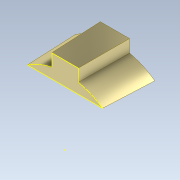
# Autodesk Inventor part: Capstonradialdisc_Aufmass
Saved by Autodesk Inventor 2022 (Build 260153000, 153)
## iProperties
Created: 2022-03-11
Part Number: Capstonradialdisc_Aufmass
Material: Generisch
Document SubType Name: Modeling
Designer: 123St
Density: 1 g/cm^3
Appearance: Gold - Metall
Author: 123St
Autodesk Inventor part; units mm, degrees
ref_plane "YZ Plane" through (0, 0, 0) normal (1, 0, 0) x (0, 1, 0)
ref_plane "XZ Plane" through (0, 0, 0) normal (0, 1, 0) x (-1, 0, 0)
ref_plane "XY Plane" through (0, 0, 0) normal (0, 0, 1) x (1, 0, 0)
sketch "Skizze1" plane through (0, 0, 0) normal (0, 0, 1) x (1, 0, 0)
  line L0 (-4, 23.3) -> (4, 23.3)
  line L1 (4, 23.3) -> (4, 20)
  line L2 (-4, 20) -> (-4, 23.3)
  line L3 (-4, 23.3) -> (4, 20) construction
  line L4 (4, 23.3) -> (-4, 20) construction
  line L5 (0, 152) -> (0, -72) projected
  line L6 (4, 20) -> (4, 19.5959)
  line L7 (-4, 20) -> (-4, 19.5959)
  arc A0 (-4, 19.5959) -> (4, 19.5959) centre (0, 0) ccw
  line L8 (-168, 0) -> (168, 0) projected
  line L9 (-35, 0) -> (-105, 0) construction
  line L10 (-35, -3) -> (-105, -3)
  line L11 (-105, 3) -> (-35, 3)
  arc A1 (-35, -3) -> (-35, 3) centre (-35, 0) ccw
  arc A2 (-105, 3) -> (-105, -3) centre (-105, 0) ccw
  arc A3 (-38.9589, -9.0666) -> (38.9589, -9.0666) centre (0, 0) ccw
  line L12 (-38.9589, -9.0666) -> (-119.657, -9.0666)
  line L13 (38.9589, -9.0666) -> (119.657, -9.0666)
  arc A4 (119.657, -9.0666) -> (-119.657, -9.0666) centre (0, 0) ccw
  arc A5 (-33.4838, 10.6223) -> (-31.1877, 16.1656) centre (-32.3358, 13.3939) ccw
  line L14 (-95.8593, 42.9534) -> (-31.1877, 16.1656)
  line L15 (-32.3358, 13.3939) -> (-97.0074, 40.1818) construction
  arc A6 (-95.8593, 42.9534) -> (-98.1554, 37.4101) centre (-97.0074, 40.1818) ccw
  line L16 (-33.4838, 10.6223) -> (-98.1554, 37.4101)
  arc A7 (-26.8701, 22.6274) -> (-22.6274, 26.8701) centre (-24.7487, 24.7487) ccw
  line L17 (-72.1249, 76.3675) -> (-22.6274, 26.8701)
  line L18 (-24.7487, 24.7487) -> (-74.2462, 74.2462) construction
  arc A8 (-72.1249, 76.3675) -> (-76.3675, 72.1249) centre (-74.2462, 74.2462) ccw
  line L19 (-26.8701, 22.6274) -> (-76.3675, 72.1249)
  arc A9 (-16.1656, 31.1877) -> (-10.6223, 33.4838) centre (-13.3939, 32.3358) ccw
  line L20 (-37.4101, 98.1554) -> (-10.6223, 33.4838)
  line L21 (-13.3939, 32.3358) -> (-40.1818, 97.0074) construction
  arc A10 (-37.4101, 98.1554) -> (-42.9534, 95.8593) centre (-40.1818, 97.0074) ccw
  line L22 (-16.1656, 31.1877) -> (-42.9534, 95.8593)
  arc A11 (-3, 35) -> (3, 35) centre (0, 35) ccw
  line L23 (3, 105) -> (3, 35)
  line L24 (0, 35) -> (0, 105) construction
  arc A12 (3, 105) -> (-3, 105) centre (0, 105) ccw
  line L25 (-3, 35) -> (-3, 105)
  arc A13 (10.6223, 33.4838) -> (16.1656, 31.1877) centre (13.3939, 32.3358) ccw
  line L26 (42.9534, 95.8593) -> (16.1656, 31.1877)
  line L27 (13.3939, 32.3358) -> (40.1818, 97.0074) construction
  arc A14 (42.9534, 95.8593) -> (37.4101, 98.1554) centre (40.1818, 97.0074) ccw
  line L28 (10.6223, 33.4838) -> (37.4101, 98.1554)
  arc A15 (22.6274, 26.8701) -> (26.8701, 22.6274) centre (24.7487, 24.7487) ccw
  line L29 (76.3675, 72.1249) -> (26.8701, 22.6274)
  line L30 (24.7487, 24.7487) -> (74.2462, 74.2462) construction
  arc A16 (76.3675, 72.1249) -> (72.1249, 76.3675) centre (74.2462, 74.2462) ccw
  line L31 (22.6274, 26.8701) -> (72.1249, 76.3675)
  arc A17 (31.1877, 16.1656) -> (33.4838, 10.6223) centre (32.3358, 13.3939) ccw
  line L32 (98.1554, 37.4101) -> (33.4838, 10.6223)
  line L33 (32.3358, 13.3939) -> (97.0074, 40.1818) construction
  arc A18 (98.1554, 37.4101) -> (95.8593, 42.9534) centre (97.0074, 40.1818) ccw
  line L34 (31.1877, 16.1656) -> (95.8593, 42.9534)
  arc A19 (35, 3) -> (35, -3) centre (35, 0) ccw
  line L35 (105, -3) -> (35, -3)
  line L36 (35, 0) -> (105, 0) construction
  arc A20 (105, -3) -> (105, 3) centre (105, 0) ccw
  line L37 (35, 3) -> (105, 3)
  line L38 (-55.3007, 11) -> (-101.4947, 30.1342)
  line L39 (-101.4947, 30.1342) -> (-105.3007, 11)
  line L40 (-105.3007, 11) -> (-55.3007, 11)
  line L41 (-82.1538, 66.7832) -> (-93.0127, 50.5755)
  line L42 (-46.8426, 31.3838) -> (-82.1538, 66.7832)
  line L43 (-93.0127, 50.5755) -> (-46.8426, 31.3838)
  line L44 (-50.2273, 93.2012) -> (-66.4754, 82.403)
  line L45 (-31.2084, 46.9597) -> (-50.2273, 93.2012)
  line L46 (-66.4754, 82.403) -> (-31.2084, 46.9597)
  line L47 (-10.6061, 105.3411) -> (-29.7544, 101.6067)
  line L48 (-10.7931, 55.3415) -> (-10.6061, 105.3411)
  line L49 (-29.7544, 101.6067) -> (-10.7931, 55.3415)
  line L50 (30.6399, 101.3432) -> (11.525, 105.2446)
  line L51 (11.2756, 55.2452) -> (30.6399, 101.3432)
  line L52 (11.525, 105.2446) -> (11.2756, 55.2452)
  line L53 (67.192, 81.8198) -> (51.0387, 92.7593)
  line L54 (31.617, 46.6855) -> (67.192, 81.8198)
  line L55 (51.0387, 92.7593) -> (31.617, 46.6855)
  line L56 (93.4505, 49.7619) -> (82.7335, 66.0637)
  line L57 (47.1147, 30.9738) -> (93.4505, 49.7619)
  line L58 (82.7335, 66.0637) -> (47.1147, 30.9738)
  line L59 (105.3927, 10.0807) -> (101.7538, 29.2473)
  line L60 (55.3946, 10.517) -> (105.3927, 10.0807)
  line L61 (101.7538, 29.2473) -> (55.3946, 10.517)
  point P0 (0, 21.65)
  point P1 (-70, 0)
  point P2 (-64.6716, 26.7878)
  point P3 (-49.4975, 49.4975)
  point P4 (-26.7878, 64.6716)
  point P5 (0, 70)
  point P6 (26.7878, 64.6716)
  point P7 (49.4975, 49.4975)
  point P8 (64.6716, 26.7878)
  point P9 (70, 0)
  dimension "d2" = 8
  dimension "d3" = 0
  dimension "d4" = 3.3
  dimension "d7" = 70
  dimension "d8" = 3
  dimension "d9" = 70
  dimension "d12" = 180
  dimension "d18" = 120
  dimension "d19" = 40
  dimension "d21" = 8
  dimension "d22" = 8
  dimension "d23" = 50
  dimension "d24" = 50
  dimension "d27" = 158
  constraints: 138 end point, 42 point on circle, 21 centre point, 5 parallel, 4 coincident, 4 point on line, 4 tangent, 3 midpoint, 2 horizontal, 1 perpendicular, 1 vertical, 147 other
  measures "d2" distance of L0.start L0.end
  measures "d3" distance from line of L5 point (0, 21.65)
  measures "d4" distance of L0.end L1.end
  measures "d7" distance of L11.start L11.end
  measures "d8" radius of A1
  measures "d9" distance of point (0, 0) point (-70, 0)
  measures "d18" radius of A4
  measures "d19" radius of A3
  measures "d21" distance between parallel lines of L11 L40
  measures "d22" distance between parallel lines of L16 L38
  measures "d23" distance of L39.end L38.start
  measures "d24" distance of L38.start L38.end
extrude "Extrusion1" add sketch "Skizze1" along normal blind 15 contours L2 L7 A0 L8 A1 L11 A2 A4 L5 A12 L25 A11 L0 | L5 A11 L23 A12 A4 L8 A20 L37 A19 A0 L6 L1 L0 | A0 L8 A19 L35 A20 A4 L13 A3 L5 | L5 A3 L12 A4 L8 A2 L10 A1 A0
fillet "Rundung1" radius 15 2 edges at (-38.9589, -9.0666, 7.5) (38.9589, -9.0666, 7.5)
fillet "Rundung2" radius 5 2 edges at (119.657, -9.0666, 7.5) (-119.657, -9.0666, 7.5)
sketch "Skizze2" plane through (49.455, -9.0666, 0) normal (0, -1, 0) x (1, 0, 0)
  circle A0 centre (62.4699, 2.5) radius 1
  line L0 (0, 0) -> (65.4731, 0) projected
  circle A1 centre (-161.38, 12.5) radius 1
  line L1 (-164.3831, 15) -> (-98.91, 15) projected
  line L2 (-169.38, 15) -> (-169.38, 0) projected
  line L3 (70.4699, 0) -> (70.4699, 15) projected
  point P0 (-49.455, 0)
  dimension "d29" = 2.5
  dimension "d30" = 2
  dimension "d31" = 2.5
  dimension "d32" = 2
  dimension "d33" = 8
  dimension "d34" = 8
  constraints: 2 centre point
  measures "d29" distance from line of L0 A0.centre
  measures "d30" diameter of A0
  measures "d31" distance from line of L1 A1.centre
  measures "d32" diameter of A1
  measures "d33" distance from line of L2 A1.centre
  measures "d34" distance from line of L3 A0.centre
extrude "Extrusion2" cut sketch "Skizze2" against normal blind 15
fillet "Rundung3" radius 2 16 edges at (-101.4947, 30.1342, 7.5) (-105.3007, 11, 7.5) (-93.0127, 50.5755, 7.5) (-66.4754, 82.403, 7.5) (-10.6061, 105.3411, 7.5) (-50.2273, 93.2012, 7.5) (-82.1538, 66.7832, 7.5) (-29.7544, 101.6067, 7.5) (30.6399, 101.3432, 7.5) (11.525, 105.2446, 7.5) (67.192, 81.8198, 7.5) (51.0387, 92.7593, 7.5) (93.4505, 49.7619, 7.5) (82.7335, 66.0637, 7.5) (101.7538, 29.2473, 7.5) (105.3927, 10.0807, 7.5)
sketch "Skizze3" plane through (0, 0, 15) normal (0, 0, 1) x (1, 0, 0)
  point P0 (0, 0)
sketch "Skizze4" plane through (0, 0, 15) normal (0, 0, 1) x (1, 0, 0)
  arc A0 (-4, 19.5959) -> (4, 19.5959) centre (0, 0) ccw projected
  line L0 (-4, 19.5959) -> (-4, 23.3) projected
  line L1 (-4, 23.3) -> (4, 23.3) projected
  line L2 (4, 23.3) -> (4, 19.5959) projected
  line L3 (-11.3027, 16.5) -> (11.3027, 16.5)
  circle A1 centre (0, 0) radius 20 construction
  line L4 (0, 20) -> (0, 0) construction
  dimension "d38" = 3.5
  constraints: 4 end point, 4 point on circle, 1 centre point, 1 coincident, 1 horizontal, 1 vertical
  measures "d38" distance from line of L3 L4.start
extrude "Extrusion3" add sketch "Skizze4" against normal up to surface (15 mm away) separate body contours L0 L1 L2 A0 L3
delete faces "Fläche löschen1" heal no whole lump yes faces at (104.9716, 12.1826, 5)
sketch "Skizze5" plane through (11.3027, 16.5, 0) normal (0, 0, -1) x (-1, 0, 0)
  line L0 (15.3027, 3.0959) -> (15.3027, 6.8) construction
  line L1 (15.3027, 6.8) -> (7.3027, 6.8) construction
  line L2 (7.3027, 6.8) -> (7.3027, 3.0959) construction
  arc A0 (7.3027, 3.0959) -> (0, 0) centre (11.3027, -16.5) ccw construction
  line L3 (0, 0) -> (22.6053, 0) construction
  arc A1 (22.6053, 0) -> (15.3027, 3.0959) centre (11.3027, -16.5) ccw construction
  line L4 (6.9027, 7.2) -> (15.7027, 7.2)
  line L5 (15.7027, 7.2) -> (15.7027, 3.4198)
  arc A2 (23.2989, 0) -> (15.7027, 3.4198) centre (11.3027, -16.5) ccw
  arc A3 (6.9027, 3.4198) -> (-0.6936, 0) centre (11.3027, -16.5) ccw
  line L6 (6.9027, 3.4198) -> (6.9027, 7.2)
  line L7 (-0.6936, 0) -> (23.2989, 0)
  dimension "d41" = 0.4
  dimension "d42" = 0.4
  dimension "d43" = 0.4
  dimension "d44" = 0.4
  constraints: 8 end point, 4 point on circle, 2 centre point, 1 collinear, 1 horizontal, 1 parallel, 1 other
  measures "d41" distance between parallel lines of L1 L4
  measures "d42" distance between parallel lines of L2 L6
  measures "d43" radial gap between concentric circles of A3 A0
  measures "d44" radial gap between concentric circles of A2 A1
sketch "Skizze6" plane through (0, 0, 15) normal (0, 0, 1) x (1, 0, 0)
  line L0 (4, 23.3) -> (-4, 23.3) projected
  line L1 (-4, 23.3) -> (-4, 19.5959) projected
  arc A0 (-4, 19.5959) -> (-11.3027, 16.5) centre (0, 0) ccw projected
  line L2 (-11.3027, 16.5) -> (11.3027, 16.5) projected
  arc A1 (11.3027, 16.5) -> (4, 19.5959) centre (0, 0) ccw projected
  line L3 (4, 19.5959) -> (4, 23.3) projected
loft "Erhebung1" add profiles "Skizze5" bodies 2 section 1 edges at (0, 23.3, 15) (-4, 21.448, 15) (-7.8063, 18.4136, 15) (0, 16.5, 15) (7.8063, 18.4136, 15) (4, 21.448, 15)
equation "\"d42\" = d41"
equation "\"d43\" = d42"
